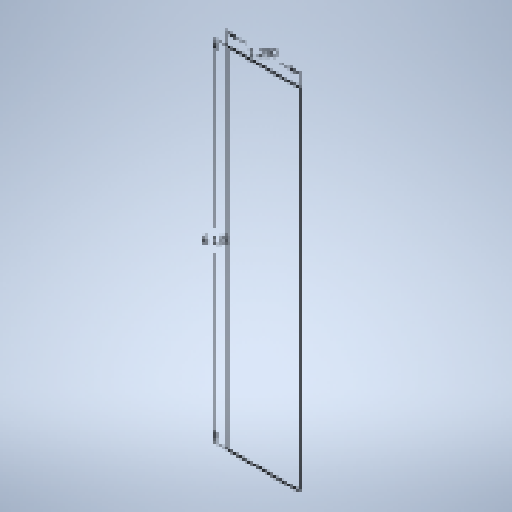
# Autodesk Inventor part: Side Plate
Saved by Autodesk Inventor 2023.4 (Build 274418000, 418)
## iProperties
Created: 2024-05-08
Part Number: Side Plate
Material: UHMW, White
Document SubType Name: Modeling
Designer: Nathan Cai
Mass: 27.3924 g
Surface Area: 114.656 cm^2
Volume: 29.1409 cm^3
Density: 0.94 g/cm^3
Appearance: Smooth - White
Author: Nathan Cai
Autodesk Inventor part; units mm, degrees
ref_plane "YZ Plane" through (0, 0, 0) normal (1, 0, 0) x (0, 1, 0)
ref_plane "XZ Plane" through (0, 0, 0) normal (0, 1, 0) x (-1, 0, 0)
ref_plane "XY Plane" through (0, 0, 0) normal (0, 0, 1) x (1, 0, 0)
sketch "Sketch1" plane through (0, 0, 0) normal (0, 0, 1) x (1, 0, 0)
  line L0 (0, 0) -> (-31.75, 0)
  line L1 (-31.75, 0) -> (-31.75, 155.575)
  line L2 (-31.75, 155.575) -> (0, 155.575)
  line L3 (0, 155.575) -> (0, 0)
  circle A0 centre (-53.975, 55.5625) radius 9.525 construction
  line L4 (-62.4238, 59.9607) -> (-12.6501, 155.575)
  point P0 (-31.75, 118.8844)
  dimension "d2" = 19.05
  dimension "d0" = 31.75
  dimension "d1" = 155.575
  dimension "d3" = 53.975
  dimension "d4" = 55.5625
  dimension "d5" = 27.5
  constraints: 10 end point, 2 parallel, 1 horizontal, 1 perpendicular, 1 point on line, 4 other
  measures "d0" distance of L1.end L2.end
  measures "d1" distance of L0.end L1.end
  measures "d3" distance from line of L3 point (-53.975, 55.562)
  measures "d4" distance from line of L0 point (-53.975, 55.562)
  measures "d5" angle of L3 L4
extrude "Extrusion1" add sketch "Sketch1" along normal blind 6.35 contours L0 L1 L4 L2 L3
body "Solid1"
